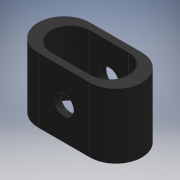
# Autodesk Inventor part: silicon_tube
Saved by Autodesk Inventor 2017 (Build 210142000, 142)
## iProperties
Created: 2018-04-08
Part Number: silicon_tube
Material: Rubber, Silicone
Document SubType Name: Modeling
Designer: Roland
Density: 1.25 g/cm^3
Appearance: Rubber - Black
Author: Roland
Autodesk Inventor part; units mm, degrees
ref_plane "YZ Plane" through (0, 0, 0) normal (1, 0, 0) x (0, 1, 0)
ref_plane "XZ Plane" through (0, 0, 0) normal (0, 1, 0) x (-1, 0, 0)
ref_plane "XY Plane" through (0, 0, 0) normal (0, 0, 1) x (1, 0, 0)
sketch "Sketch1" plane through (0, 0, 0) normal (0, 0, 1) x (1, 0, 0)
  line L0 (-4, 0) -> (4, 0) construction
  line L1 (-4, -4) -> (4, -4)
  line L2 (4, 4) -> (-4, 4)
  arc A0 (-4, 4) -> (-4, -4) centre (-4, 0) ccw
  arc A1 (4, -4) -> (4, 4) centre (4, 0) ccw
  line L3 (-3, 0) -> (3, 0) construction
  line L4 (-3, -3) -> (3, -3)
  line L5 (3, 3) -> (-3, 3)
  arc A2 (-3, 3) -> (-3, -3) centre (-3, 0) ccw
  arc A3 (3, -3) -> (3, 3) centre (3, 0) ccw
  point P0 (0, 0)
  constraints: 16 end point, 8 point on circle, 8 tangent, 4 centre point, 2 midpoint, 2 parallel, 1 horizontal, 1 point on line
extrude "Extrusion1" add sketch "Sketch1" along normal blind 10
sketch "Sketch2" plane through (-4, 4, 0) normal (0, 1, 0) x (1, 0, 0)
  point P0 (4, 0)
  point P1 (4, -5)
hole "Hole1" at (0, 4, 5) direction (0, -1, 0) diameter 3 end through all
body "Solid1"
